Autodesk Inventor part; units mm, degrees
(part 2 of 2)
sketch "スケッチ16" plane through (0, 0, 3) normal (0, 0, 1) x (1, 0, 0)
  line L0 (-24.4121, 84.9889) -> (-12.8854, 81.652) projected
  arc A0 (-12.8854, 81.652) -> (-13.4416, 79.7309) centre (-13.1635, 80.6914) ccw projected
  line L1 (-13.4416, 79.7309) -> (-16.2223, 70.1253) projected
  arc A1 (-16.2223, 70.1253) -> (-16.7785, 68.2042) centre (-16.5004, 69.1647) ccw projected
  line L2 (-16.7785, 68.2042) -> (-28.3052, 71.5411) projected
  arc A2 (-28.3052, 71.5411) -> (-27.749, 73.4622) centre (-28.0271, 72.5017) ccw projected
  line L3 (-27.749, 73.4622) -> (-24.9683, 83.0678) projected
  arc A3 (-24.9683, 83.0678) -> (-24.4121, 84.9889) centre (-24.6902, 84.0284) ccw projected
  circle A4 centre (-11.9503, 74.0939) radius 1.5 projected
  circle A5 centre (-6.1515, 120.3493) radius 1.5 projected
  circle A6 centre (-24.1421, 119.7668) radius 1.5 projected
  circle A7 centre (-29.2403, 79.0993) radius 1.5 projected
  arc A8 (-9.3765, 127.2485) -> (-9.3118, 125.2496) centre (-9.3441, 126.249) ccw projected
  line L4 (-9.3118, 125.2496) -> (-8.9882, 115.2548) projected
  arc A9 (-8.9882, 115.2548) -> (-8.9234, 113.2558) centre (-8.9558, 114.2553) ccw projected
  line L5 (-8.9234, 113.2558) -> (-20.9172, 112.8675) projected
  arc A10 (-20.9172, 112.8675) -> (-20.9819, 114.8665) centre (-20.9495, 113.867) ccw projected
  line L6 (-20.9819, 114.8665) -> (-21.3055, 124.8612) projected
  arc A11 (-21.3055, 124.8612) -> (-21.3702, 126.8602) centre (-21.3378, 125.8607) ccw projected
  line L7 (-21.3702, 126.8602) -> (-9.3765, 127.2485) projected
  circle A12 centre (55.4, 111) radius 1.25 projected
  circle A13 centre (25, 100.25) radius 1.5 projected
  circle A14 centre (0, 66.75) radius 1.5 projected
  circle A15 centre (25, 66.75) radius 1.5 projected
  circle A16 centre (0, 100.25) radius 1.5 projected
  circle A17 centre (55.3, 64) radius 1.6 projected
  line L8 (23, 137) -> (23, 140) projected
  arc A18 (23, 140) -> (25, 140) centre (24, 140) ccw projected
  line L9 (25, 140) -> (29, 140) projected
  arc A19 (29, 140) -> (29.866, 138.5) centre (29, 139) ccw projected
  arc A20 (29.866, 138.5) -> (29, 137) centre (29, 138) ccw projected
  line L10 (29, 137) -> (25, 137) projected
  arc A21 (25, 137) -> (23, 137) centre (24, 137) ccw projected
  line L11 (51, 140) -> (55, 140) projected
  arc A22 (55, 140) -> (57, 140) centre (56, 140) ccw projected
  line L12 (57, 140) -> (57, 137) projected
  arc A23 (57, 137) -> (55, 137) centre (56, 137) ccw projected
  line L13 (55, 137) -> (51, 137) projected
  arc A24 (51, 137) -> (50.134, 138.5) centre (51, 138) ccw projected
  arc A25 (50.134, 138.5) -> (51, 140) centre (51, 139) ccw projected
  line L14 (37, 137) -> (37, 140) projected
  arc A26 (37, 140) -> (39, 140) centre (38, 140) ccw projected
  line L15 (39, 140) -> (43, 140) projected
  arc A27 (43, 140) -> (43.866, 138.5) centre (43, 139) ccw projected
  arc A28 (43.866, 138.5) -> (43, 137) centre (43, 138) ccw projected
  line L16 (43, 137) -> (39, 137) projected
  arc A29 (39, 137) -> (37, 137) centre (38, 137) ccw projected
  circle A30 centre (-12.461, 47.5151) radius 1.2295 projected
  circle A31 centre (-34.1345, 137.9496) radius 1.2295 projected
  circle A32 centre (-19.3858, 140.684) radius 1.2295 projected
  circle A33 centre (-30.5132, 56.1243) radius 1.2295 projected
  circle A34 centre (-1.5, 36) radius 1.6 projected
  circle A35 centre (-1.5, 144) radius 1.6 projected
  circle A36 centre (30, 16) radius 1.6 projected
  circle A37 centre (30, 124) radius 1.6 projected
  line L17 (62.5, 150) -> (-47.5, 150) projected
  line L18 (-47.5, 150) -> (-47.5, 10) projected
  line L19 (-47.5, 10) -> (62.5, 10) projected
  line L20 (62.5, 10) -> (62.5, 150) projected
  arc A38 (59.9998, 139.9632) -> (56.3191, 143.9873) centre (56, 140) ccw
  arc A39 (-34.7386, 55.9373) -> (-33.6099, 53.2435) centre (-30.5132, 56.1243) ccw
  arc A40 (-34.9519, 142.0993) -> (-38.3598, 137.7626) centre (-34.1345, 137.9496) ccw
  line L21 (-20.2327, 144.9986) -> (-34.9519, 142.0993)
  line L22 (-38.3598, 137.7626) -> (-34.7386, 55.9373)
  line L23 (6.1596, 12.0145) -> (29.4894, 10.0218)
  line L24 (59.2998, 63.9632) -> (59.9998, 139.9632)
  arc A41 (-1.133, 148.5853) -> (-2.389, 148.5133) centre (-1.5, 144) ccw
  line L25 (-20.2327, 144.9986) -> (-2.389, 148.5133)
  line L26 (-1.133, 148.5853) -> (56.3191, 143.9873)
  circle A42 centre (21.5, 22) radius 1.6 projected
  arc A43 (18.5, 15) -> (18.5, 17) centre (18.5, 16) ccw projected
  line L27 (18.5, 15) -> (6.5, 15) projected
  arc A44 (6.5, 17) -> (6.5, 15) centre (6.5, 16) ccw projected
  line L28 (6.5, 17) -> (6.5, 27) projected
  arc A45 (6.5, 29) -> (6.5, 27) centre (6.5, 28) ccw projected
  line L29 (6.5, 29) -> (18.5, 29) projected
  arc A46 (18.5, 27) -> (18.5, 29) centre (18.5, 28) ccw projected
  line L30 (18.5, 27) -> (18.5, 17) projected
  circle A47 centre (3.5, 22) radius 1.6 projected
  arc A48 (3.5713, 13.2755) -> (6.5, 12) centre (6.5, 16) ccw
  line L31 (-33.6099, 53.2435) -> (3.5713, 13.2755)
  circle A49 centre (43.2987, 57.3213) radius 1.25 projected
  circle A50 centre (43.3013, 22.6802) radius 1.25 projected
  line L32 (35.3, 23.7) -> (33.3, 23.7) projected
  arc A51 (33.3, 23.7) -> (33.3, 56.3) centre (33.3, 40) ccw projected
  line L33 (33.3, 56.3) -> (35.3, 56.3) projected
  circle A52 centre (13.3, 39.9985) radius 1.25 projected
  circle A53 centre (55.4, 87) radius 1.2295 projected
  arc A54 (45.0562, 20.5259) -> (42.136, 25.2027) centre (43.3013, 22.6802) ccw
  arc A55 (29.4894, 10.0218) -> (33.7894, 11.3481) centre (30, 16) ccw
  line L34 (33.7894, 11.3481) -> (45.0562, 20.5259)
  arc A56 (56.9267, 60.3457) -> (59.2998, 63.9632) centre (55.3, 64) ccw
  arc A57 (42.1337, 54.7983) -> (44.4288, 54.7825) centre (43.2987, 57.3213) ccw
  line L35 (56.9267, 60.3457) -> (44.4288, 54.7825)
  arc A58 (35.3, 23.7) -> (42.136, 25.2027) centre (35.3, 40) ccw
  arc A59 (42.1337, 54.7983) -> (35.3, 56.3) centre (35.3, 40) ccw
  point P0 (0, 0)
  dimension "d160" = 3
  dimension "d161" = 3
  dimension "d163" = 3
  dimension "d164" = 4
  dimension "d185" = 4
  dimension "d206" = 4
  dimension "d207" = 6
  dimension "d209" = 12
  dimension "d210" = 16.3
  constraints: 50 centre point, 23 point on circle, 18 end point, 17 tangent, 4 coincident, 1 collinear, 1 concentric
  measures "d160" radial gap between concentric circles of A33 A39
  measures "d161" radial gap between concentric circles of A31 A40
  measures "d163" radial gap between concentric circles of A35 A41
  measures "d164" radius of A38
  measures "d185" radius of A48
  measures "d206" distance from line of L24 A17.centre
  measures "d207" distance from line of L23 A36.centre
  measures "d209" diameter of A55
  measures "d210" radius of A58
extrude "型抜き" cut sketch "スケッチ16" against normal through all contours A20 A19 | L8 A18 L9 A19 A20 L10 A21 | A25 A24 | L11 A22 L12 A23 L13 A24 A25 | A28 A27 | L14 A26 L15 A27 A28 L16 A29 | A55 L23 A48 L31 A39 L22 A40 L21 L25 A41 L26 A38 L24 A56 L35 A57 A59 L33 A51 L32 A58 A54 L34 | A42 | L27 A44 L28 A45 L29 A46 L30 A43 | A47 | A49 | A50 | A52 | A53 keep common part
equation "\"d2\" = d3"
equation "\"d5\" = d2"
equation "\"d8\" = d7"
